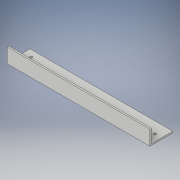
# Autodesk Inventor part: angle iron with  holes 2
Saved by Autodesk Inventor 2018 (Build 220112000, 112)
## iProperties
Created: 2019-02-23
Part Number: angle iron with  holes 2
Material: Generic
Document SubType Name: Modeling
Designer: s-2513225
Density: 1 g/cm^3
Appearance: Default
Author: s-2513225
Autodesk Inventor part; units mm, degrees
ref_plane "YZ Plane" through (0, 0, 0) normal (1, 0, 0) x (0, 1, 0)
ref_plane "XZ Plane" through (0, 0, 0) normal (0, 1, 0) x (-1, 0, 0)
ref_plane "XY Plane" through (0, 0, 0) normal (0, 0, 1) x (1, 0, 0)
sketch "Sketch1" plane through (0, 0, 0) normal (0, 1, 0) x (-1, 0, 0)
  line L0 (0, 0) -> (279.4, 0)
  line L1 (279.4, 0) -> (279.4, -44.577)
  line L2 (279.4, -44.577) -> (0, -44.577)
  line L3 (0, -44.577) -> (0, 0)
  dimension "d0" = 279.4
  dimension "d1" = 44.577
  constraints: 8 end point, 2 parallel, 1 horizontal, 1 perpendicular
  measures "d0" distance of L1.end L2.end
  measures "d1" distance of L0.end L1.end
extrude "Extrusion1" add sketch "Sketch1" along normal blind 3.175
sketch "Sketch2" plane through (0, 3.175, 0) normal (0, 1, 0) x (1, 0, 0)
  line L0 (-279.4, 0) -> (0, 0) projected
  line L1 (-279.4, 0) -> (0, 0)
  line L2 (0, 0) -> (0, 3.175)
  line L3 (0, 3.175) -> (-279.4, 3.175)
  line L4 (-279.4, 3.175) -> (-279.4, 0)
  dimension "d4" = 279.4
  dimension "d5" = 3.175
  constraints: 8 end point, 2 parallel, 1 horizontal, 1 perpendicular
  measures "d4" distance of L3.end L2.end
  measures "d5" distance of L2.end L1.end
extrude "Extrusion2" add sketch "Sketch2" along normal blind 25.4
sketch "Sketch3" plane through (0, 3.175, 0) normal (0, 1, 0) x (1, 0, 0)
  line L0 (0, 3.175) -> (0, 44.577) construction
  line L1 (0, 44.577) -> (-279.4, 44.577) construction
  line L2 (-139.7, 44.577) -> (-139.7, 3.175) construction
  line L3 (-279.4, 44.577) -> (-248.5898, 44.577) construction
  line L4 (-248.5898, 44.577) -> (-248.5898, 20.574) construction
  circle A0 centre (-248.5898, 20.574) radius 2.5797
  line L5 (-248.5898, 20.574) -> (-264.1372, 31.5822) construction
  circle A1 centre (-264.1372, 31.5822) radius 2.5797
  point P0 (0, 0)
  constraints: 8 end point, 2 centre point, 2 coincident, 1 midpoint, 1 vertical
extrude "Extrusion3" cut sketch "Sketch3" against normal blind 25.4
sketch "Sketch4" plane through (0, 3.175, 0) normal (0, 1, 0) x (1, 0, 0)
  line L0 (0, 3.175) -> (0, 44.577) construction
  line L1 (0, 44.577) -> (-279.4, 44.577) construction
  line L2 (0, 23.1034) -> (-12.7, 23.1034) construction
  line L3 (-12.7, 44.577) -> (-12.7, 22.352) construction
  circle A0 centre (-12.7, 22.352) radius 2.5797
  point P0 (0, 0)
  dimension "d26" = 12.7
  dimension "d27" = 22.225
  dimension "d28" = 5.1594
  constraints: 4 end point, 2 point on line, 1 centre point, 1 coincident, 1 parallel, 1 vertical
  measures "d26" distance of L2.start L2.end
  measures "d27" distance of L3.start L3.end
  measures "d28" diameter of A0
extrude "Extrusion4" cut sketch "Sketch4" against normal blind 25.4
body "Solid1"
